Autodesk Fusion 360 part; units mm, degrees
note: some values were not read from the file. Set by a fixed rule: which face or edge a step refers to.
(part 2 of 2)
sketch "Sketch45" plane through (0, 0, 5) normal (0, 0, 1) x (-1, 0, 0)
  line L0 (20, -135) -> (22, -135)
  line L1 (22, -135) -> (22, -137)
  line L2 (22, -137) -> (2, -137)
  line L3 (2, -137) -> (2, -147.75)
  line L4 (2, -147.75) -> (75, -147.75)
  line L5 (75, -147.75) -> (80, -142.75)
  line L6 (80, -142.75) -> (80, -130)
  line L7 (80, -130) -> (78, -130)
  line L8 (78, -130) -> (78, -120)
  line L9 (78, -120) -> (80, -120)
  line L10 (80, -120) -> (80, -107.25)
  line L11 (80, -107.25) -> (75, -102.25)
  line L12 (75, -102.25) -> (2, -102.25)
  line L13 (2, -102.25) -> (2, -113)
  line L14 (2, -113) -> (22, -113)
  line L15 (22, -113) -> (22, -115)
  line L16 (22, -115) -> (20, -115)
  line L17 (20, -115) -> (20, -135)
  line L18 (22, -115) -> (20, -115)
  line L19 (20, -115) -> (20, -135)
  line L20 (20, -135) -> (22, -135)
  line L21 (22, -135) -> (22, -115)
  constraint horizontal L18
  constraint vertical L19
  constraint horizontal L20
  constraint vertical L21
  constraint coincident L0.start L17.end
  constraint coincident L15.end L16.start
sketch "Sketch46" plane through (0, 0, 5) normal (0, 0, 1) x (-1, 0, 0)
  line L0 (20, -135) -> (22, -135)
  line L1 (22, -135) -> (22, -137)
  line L2 (22, -137) -> (2, -137)
  line L3 (2, -137) -> (2, -147.75)
  line L4 (2, -147.75) -> (75, -147.75)
  line L5 (75, -147.75) -> (80, -142.75)
  line L6 (80, -142.75) -> (80, -130)
  line L7 (80, -130) -> (78, -130)
  line L8 (78, -130) -> (78, -120)
  line L9 (78, -120) -> (80, -120)
  line L10 (80, -120) -> (80, -107.25)
  line L11 (80, -107.25) -> (75, -102.25)
  line L12 (75, -102.25) -> (2, -102.25)
  line L13 (2, -102.25) -> (2, -113)
  line L14 (2, -113) -> (22, -113)
  line L15 (22, -113) -> (22, -115)
  line L16 (22, -115) -> (20, -115)
  line L17 (20, -115) -> (20, -135)
extrude "Extrude62" add sketch "Sketch45" along normal blind 14.54 contours L0 L16 L17 L18 L19 L20 L21 bodies 6
fillet "Fillet24" radius 10 2 edges at (-20, 115, 9.7699) (-20, 135, 9.7699) on bodies 6
